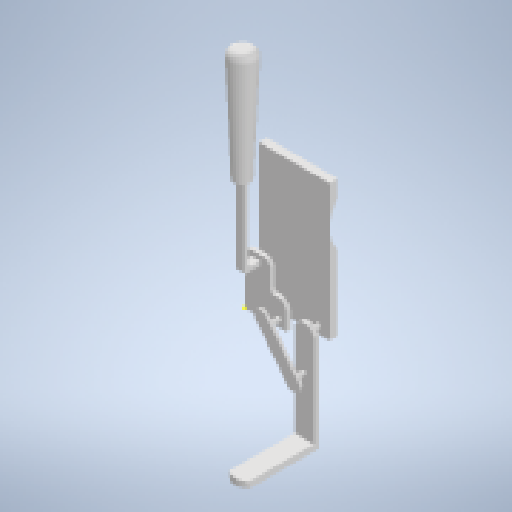
# Autodesk Inventor part: G26 P999999
Saved by Autodesk Inventor 2023 (Build 270158000, 158)
## iProperties
Created: 2023-10-24
Part Number: G26 P999999
Material: Generic
Document SubType Name: Modeling
Designer: Rajat K
Density: 1 g/cm^3
Appearance: Default
Author: Rajat K
Autodesk Inventor part; units mm, degrees
ref_plane "YZ Plane" through (0, 0, 0) normal (1, 0, 0) x (0, 1, 0)
ref_plane "XZ Plane" through (0, 0, 0) normal (0, 1, 0) x (-1, 0, 0)
ref_plane "XY Plane" through (0, 0, 0) normal (0, 0, 1) x (1, 0, 0)
sketch "Sketch1" plane through (0, 0, 0) normal (0, 0, 1) x (1, 0, 0)
  line L0 (0, 42.225) -> (0, 0)
  line L1 (0, 0) -> (22, 0)
  line L2 (22, 0) -> (22, 42.225)
  line L3 (22, 42.225) -> (0, 42.225)
  dimension "d0" = 22
  dimension "d1" = 42.225
  constraints: 8 end point, 3 perpendicular, 1 vertical
  measures "d0" distance between parallel lines of L2 L0
  measures "d1" distance between parallel lines of L1 L3
extrude "Extrusion1" add sketch "Sketch1" along normal blind 2.5
sketch "Sketch2" plane through (0, 0, 0) normal (-1, 0, 0) x (0, 0, 1)
  line L0 (2.5, 0) -> (2.5, 42.225) projected
  arc A0 (0, 23.1358) -> (0, 37.1892) centre (-8.625, 30.1625) ccw
  line L1 (0, 0) -> (0, 42.225) projected
  line L2 (0, 23.1358) -> (0, 37.1892)
  dimension "d62" = 22.25
  dimension "d63" = 0
  constraints: 2 end point, 2 point on circle, 2 point on line, 1 centre point
  measures "d62" diameter of A0
  measures "d63" distance edge to line of A0 L0
extrude "Extrusion2" cut sketch "Sketch2" against normal through all
sketch "Sketch3" plane through (0, 0, 2.5) normal (0, 0, 1) x (1, 0, 0)
  circle A0 centre (2.1436, 2.3013) radius 0.75
  point P0 (0, 0)
  dimension "d7" = 1.5
  constraints: 1 centre point
  measures "d7" diameter of A0
extrude "Extrusion3" add sketch "Sketch3" along normal blind 3
sketch "Sketch4" plane through (2.1436, 2.3013, 5.5) normal (0, 0, 1) x (1, 0, 0)
  line L0 (-2.1436, -2.3013) -> (19.8564, -2.3013) projected
  line L1 (-2.1436, -2.3013) -> (10.8564, -2.3013)
  line L2 (10.8564, -2.3013) -> (10.8564, 2.6987)
  line L3 (7.8564, 5.6987) -> (6.8564, 5.6987)
  line L4 (5.8564, 6.6987) -> (5.8564, 12.1987)
  line L5 (3.8564, 14.1987) -> (-0.1436, 14.1987)
  line L6 (-2.1436, 39.9237) -> (-2.1436, -2.3013) projected
  line L7 (-2.1436, -2.3013) -> (-2.1436, 12.1987)
  arc A0 (-0.1436, 14.1987) -> (-2.1436, 12.1987) centre (-0.1436, 12.1987) ccw
  arc A1 (5.8564, 12.1987) -> (3.8564, 14.1987) centre (3.8564, 12.1987) ccw
  arc A2 (5.8564, 6.6987) -> (6.8564, 5.6987) centre (6.8564, 6.6987) ccw
  arc A3 (10.8564, 2.6987) -> (7.8564, 5.6987) centre (7.8564, 2.6987) ccw
  point P0 (-2.1436, 14.1987)
  point P1 (-2.1436, 17.6987)
  point P2 (8.8564, -2.3013)
  dimension "d10" = 8
  dimension "d11" = 8
  dimension "d12" = 16.5
  dimension "d13" = 13
  dimension "d14" = 2
  dimension "d15" = 2
  dimension "d16" = 1
  dimension "d17" = 3
  constraints: 12 end point, 8 point on circle, 8 tangent, 4 centre point, 4 perpendicular, 4 point on line, 1 midpoint, 1 vertical
  measures "d10" distance between parallel lines of L4 L6
  measures "d11" distance from line of point (8.856, -2.301) L3
  measures "d12" distance between parallel lines of L0 L5
  measures "d13" distance between parallel lines of L2 L6
  measures "d14" radius of A0
  measures "d15" radius of A1
  measures "d16" radius of A2
  measures "d17" radius of A3
extrude "Extrusion4" add sketch "Sketch4" along normal blind 1.3
sketch "Sketch5" plane through (2.1436, 2.3013, 6.8) normal (0, 0, 1) x (1, 0, 0)
  point P0 (-2.1436, -2.3013)
sketch "Sketch6" plane through (0, 0, 2.5) normal (0, 0, 1) x (1, 0, 0)
  circle A0 centre (18.5926, 2.3013) radius 0.75
  point P0 (0, 0)
  dimension "d20" = 1.5
  constraints: 1 centre point
  measures "d20" diameter of A0
extrude "Extrusion5" add sketch "Sketch6" along normal blind 3
sketch "Sketch7" plane through (18.5926, 2.3013, 5.5) normal (0, 0, 1) x (1, 0, 0)
  circle A0 centre (0, 0) radius 0.75 projected
  line L0 (0, 0) -> (6, 0)
  line L1 (0, 0) -> (3, 0)
  line L2 (3, 0) -> (3, -30)
  line L3 (3, -30) -> (0, -30)
  line L4 (0, -0.75) -> (0, 0)
  line L5 (0, 0) -> (-3, 0)
  line L6 (-3, 0) -> (-3, -30)
  line L7 (-3, -30) -> (0, -30)
  line L8 (0, -0.75) -> (0, 0)
  arc A1 (3, 0) -> (-3, 0) centre (0, 0) ccw
  point P0 (-18.5926, -2.3013)
  point P1 (-1.5, -30)
  point P2 (0, -30)
  dimension "d23" = 3
  dimension "d24" = 3
  dimension "d25" = 30
  constraints: 18 end point, 4 parallel, 3 horizontal, 2 perpendicular, 2 point on circle, 2 tangent, 1 centre point, 1 midpoint, 1 point on line, 1 vertical alignment, 1 other
  measures "d23" distance between parallel lines of L2 L4
  measures "d24" distance between parallel lines of L4 L6
  measures "d25" distance from line of point (-1.5, -30) L5
extrude "Extrusion6" add sketch "Sketch7" along normal blind 1.5
sketch "Sketch8" plane through (2.1436, 2.3013, 6.8) normal (0, 0, 1) x (1, 0, 0)
  circle A0 centre (8.4665, -0.0248) radius 0.75
  point P0 (-2.1436, -2.3013)
  dimension "d28" = 1.5
  constraints: 1 centre point
  measures "d28" diameter of A0
extrude "Extrusion7" add sketch "Sketch8" along normal blind 3
sketch "Sketch9" plane through (2.1436, 2.3013, 6.8) normal (0, 0, 1) x (1, 0, 0)
  line L0 (0.1064, 12.6987) -> (2.6064, 12.6987)
  line L1 (2.6064, 12.6987) -> (2.6064, 11.1987)
  line L2 (2.6064, 11.1987) -> (0.1064, 11.1987)
  line L3 (0.1064, 11.1987) -> (0.1064, 12.6987)
  line L4 (3.8564, 14.1987) -> (-0.1436, 14.1987) projected
  line L5 (-2.1436, 12.1987) -> (-2.1436, -2.3013) projected
  dimension "d31" = 2.5
  dimension "d32" = 1.5
  dimension "d33" = 1.5
  dimension "d34" = 2.25
  constraints: 8 end point, 2 parallel, 1 horizontal, 1 perpendicular
  measures "d31" distance of L1.end L2.end
  measures "d32" distance of L0.end L1.end
  measures "d33" distance between parallel lines of L4 L0
  measures "d34" distance between parallel lines of L5 L3
extrude "Extrusion8" add sketch "Sketch9" along normal blind 5
sketch "Sketch10" plane through (2.25, 13.5, 6.8) normal (-1, 0, 0) x (0, 0, 1)
  point P0 (-6.8, -13.5)
sketch "Sketch11" plane through (2.25, 15, 6.8) normal (0, 1, 0) x (1, 0, 0)
  line L0 (0, -5) -> (2.5, -5) projected
  line L1 (0, 0) -> (0, -5) projected
  line L2 (2.5, -5) -> (0, -5)
  line L3 (0, -5) -> (0, -3.5)
  line L4 (0, -3.5) -> (2.5, -3.5)
  line L5 (2.5, -3.5) -> (2.5, -5)
  point P0 (-2.25, 6.8)
  dimension "d37" = 1.5
  constraints: 8 end point, 2 parallel, 1 horizontal, 1 perpendicular, 1 point on line
  measures "d37" distance of L4.end L0.end
extrude "Extrusion9" add sketch "Sketch11" along normal blind 23.5
fillet "Fillet1" radius 1 1 edges at (3.5, 13.5, 11.8)
fillet "Fillet2" radius 1 1 edges at (3.5, 15, 10.3)
sketch "Sketch12" plane through (2.25, 38.5, 6.8) normal (0, 1, 0) x (1, 0, 0)
  line L0 (2.5, -5) -> (0, -5) projected
  line L1 (1.25, -5) -> (1.25, -4.25)
  circle A0 centre (1.25, -4.25) radius 4
  point P0 (-2.25, 6.8)
  dimension "d42" = 0.75
  dimension "d43" = 8
  constraints: 2 end point, 1 centre point, 1 coincident, 1 midpoint, 1 vertical
  measures "d42" distance of L1.start L1.end
  measures "d43" diameter of A0
extrude "Extrusion10" add sketch "Sketch12" along normal blind 35
draft "FaceDraft1" angle 2.5 pull direction (0, -1, 0) faces at (7.487, 61.8333, 11.3719) fixed edges at (-0.5, 73.5, 11.05)
fillet "Fillet3" radius 2 1 edges at (-0.5, 73.5, 11.05)
sketch "Sketch13" plane through (18.5926, 2.3013, 7) normal (0, 0, 1) x (1, 0, 0)
  circle A0 centre (-7.9825, -0.0248) radius 0.75 projected
  circle A1 centre (0.0757, -10.2261) radius 0.75
  line L0 (-7.9825, -0.0248) -> (-7.5176, -0.6133)
  line L1 (-0.3892, -9.6376) -> (0.0757, -10.2261)
  point P0 (-18.5926, -2.3013)
  dimension "d49" = 1.5
  dimension "d48" = 13
  constraints: 4 end point, 1 coincident, 5 other
  measures "d48" distance of L0.start L1.end
extrude "Extrusion11" add sketch "Sketch13" along normal blind 3 contours A1
sketch "Sketch14" plane through (10.6101, 2.2765, 9.8) normal (0, 0, 1) x (1, 0, 0)
  line L0 (-2.8011, -0.2255) -> (6.8738, -12.7955)
  line L1 (10.9825, -29.9752) -> (10.9825, 0.0248) projected
  line L2 (0.3433, 2.2472) -> (9.9183, -10.1929)
  arc A0 (0.3433, 2.2472) -> (-2.8011, -0.2255) centre (-1.5459, 1.414) ccw
  arc A1 (6.8738, -12.7955) -> (9.9183, -10.1929) centre (8.1356, -11.1896) ccw
  point P0 (-10.6101, -2.2765)
  dimension "d52" = 4
  constraints: 4 end point, 4 point on circle, 2 centre point
  measures "d52" distance between parallel lines of L2 L0
extrude "Extrusion12" add sketch "Sketch14" along normal blind 1
sketch "Sketch15" plane through (18.5926, 2.3013, 7) normal (0, 0, 1) x (1, 0, 0)
  line L0 (-3, 0) -> (-3, -30) projected
  line L1 (-3, -28) -> (3, -28)
  line L2 (3, -28) -> (3, -30)
  line L3 (3, -30) -> (-3, -30)
  line L4 (-3, -30) -> (-3, -28)
  point P0 (-18.5926, -2.3013)
  dimension "d56" = 2
  constraints: 8 end point, 2 parallel, 1 horizontal, 1 perpendicular, 1 point on line
  measures "d56" distance between parallel lines of L3 L1
extrude "Extrusion13" add sketch "Sketch15" along normal blind 20
sketch "Sketch16" plane through (15.5926, -25.6987, 7) normal (0, 1, 0) x (1, 0, 0)
  line L0 (0, -20) -> (6, -20) projected
  arc A0 (0, -20) -> (6, -20) centre (3, -16.7649) ccw
  point P0 (-15.5926, 7)
  dimension "d59" = 4.412
  constraints: 2 point on circle, 1 centre point
  measures "d59" radius of A0
extrude "Extrusion14" add sketch "Sketch16" against normal blind 2
body "Solid1"
